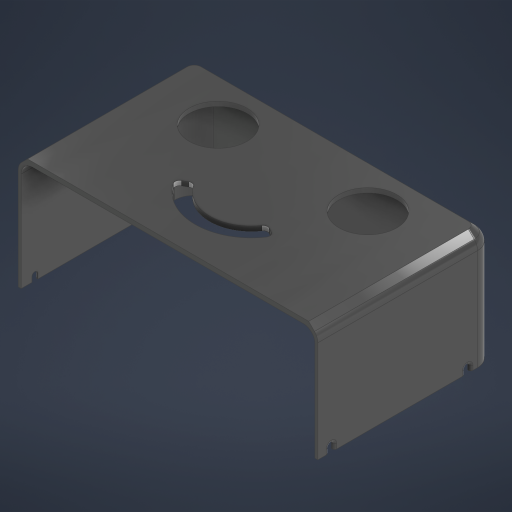
# Autodesk Inventor part: Mixer and nozzle cover
Saved by Autodesk Inventor 2024 (Build 280153000, 153)
## iProperties
Created: 2024-11-27
Part Number: Mixer and nozzle cover
Material: Generic
Document SubType Name: Modeling
Designer: Vincent Larson
Density: 1 g/cm^3
Appearance: Default
Author: Vincent Larson
## iProperties of the stored document Mixer and nozzle cover_3DPrint.ipt
Created: 2024-11-27
Part Number: Mixer and nozzle cover_3DPrint
Material: Generic
Document SubType Name: Modeling
Designer: Vincent Larson
Density: 1 g/cm^3
Appearance: Default
Author: Vincent Larson
Autodesk Inventor part; units mm, degrees
ref_plane "YZ Plane" through (0, 0, 0) normal (1, 0, 0) x (0, 1, 0)
ref_plane "XZ Plane" through (0, 0, 0) normal (0, 1, 0) x (-1, 0, 0)
ref_plane "XY Plane" through (0, 0, 0) normal (0, 0, 1) x (1, 0, 0)
sketch "Sketch1" plane through (0, 0, 0) normal (0, 1, 0) x (-1, 0, 0)
  line L0 (0, 0) -> (0, -70.91)
  line L1 (0, 0) -> (-126.245, 0)
  line L2 (-126.245, 0) -> (-126.245, -70.91)
  line L3 (-126.245, -70.91) -> (0, -70.91)
  line L4 (0, -70.91) -> (0, 0)
  line L5 (-126.245, -70.91) -> (-118.245, -70.91)
  line L6 (-118.245, -70.91) -> (-118.245, -62.91)
  circle A0 centre (-118.245, -62.91) radius 8
  line L7 (0, 0) -> (-8, 0)
  line L8 (-8, 0) -> (-8, -8)
  line L9 (-8, -8) -> (0, -8)
  line L10 (0, -8) -> (0, 0)
  circle A1 centre (-8, -62.91) radius 8
  line L11 (0.5, 0) -> (0.5, -70.91)
  circle A2 centre (-8, -62.91) radius 8.5
  line L12 (-126.245, -71.41) -> (0.5, -71.41)
  line L13 (0.5, -71.41) -> (0.5, 0)
  circle A3 centre (-118.245, -62.91) radius 8.5
  line L14 (-126.745, -70.91) -> (-126.745, 0.5)
  line L15 (-126.745, 0.5) -> (0, 0.5)
  line L16 (-8.5, 0.5) -> (0.5, 0.5)
  line L17 (0.5, 0.5) -> (0.5, -8.5)
  line L18 (0.5, -8.5) -> (-8.5, -8.5)
  line L19 (-8.5, -8.5) -> (-8.5, 0.5)
  line L20 (0.5, 0.5) -> (1.77, 0.5)
  line L21 (-126.745, -71.41) -> (-124.2953, -71.41)
  line L22 (-126.745, -69.4465) -> (-126.745, -71.41)
  circle A4 centre (-126.745, -71.41) radius 0.635
  line L23 (-127.38, -72.045) -> (1.77, -72.045)
  line L24 (1.77, -72.045) -> (1.77, 0.5)
  line L25 (1.77, 0.5) -> (-127.38, 0.5)
  line L26 (-127.38, 0.5) -> (-127.38, -72.045)
  line L27 (1.77, 0.5) -> (0.5, 0.5)
  line L28 (0.5, 0.5) -> (0.5, 3.5)
  line L29 (0.5, 3.5) -> (1.77, 3.5)
  line L30 (1.77, 3.5) -> (1.77, 0.5)
  line L31 (-126.745, 0.5) -> (-128.015, 0.5)
  line L32 (-128.015, 0.5) -> (-128.015, -72.045)
  line L33 (-128.015, -72.045) -> (-126.745, -72.045)
  line L34 (-126.745, -72.045) -> (-126.745, 0.5)
  line L35 (1.77, -71.41) -> (-128.015, -71.41)
  line L36 (-128.015, -71.41) -> (-128.015, -72.68)
  line L37 (-128.015, -72.68) -> (1.77, -72.68)
  line L38 (1.77, -72.68) -> (1.77, -71.41)
  line L39 (-126.745, 0.5) -> (-128.015, 0.5)
  line L40 (-128.015, 0.5) -> (-128.015, 3.5)
  line L41 (-128.015, 3.5) -> (-126.745, 3.5)
  line L42 (-126.745, 3.5) -> (-126.745, 0.5)
  point P0 (0.5, -62.91)
  point P1 (-8, -71.41)
  point P2 (-118.245, -71.41)
  point P3 (-126.745, -62.91)
  point P4 (-126.745, 0.5)
  point P5 (0.5, 0.5)
  point P6 (-126.745, 0.5)
  point P7 (1.77, -72.045)
  dimension "d0" = 70.91
  dimension "d1" = 126.245
  dimension "d2" = 8
  dimension "d3" = 8
  dimension "d4" = 8
  dimension "d5" = 8
  dimension "d6" = 0.5
  dimension "d7" = 0.5
  dimension "d8" = 0.5
  dimension "d9" = 0.5
  dimension "d10" = 0.5
  dimension "d11" = 0.5
  dimension "d12" = 1.27
  dimension "d13" = 1.27
  dimension "d16" = 3
  dimension "d17" = 1.27
  dimension "d18" = 1.27
  constraints: 86 end point, 18 parallel, 9 perpendicular, 8 horizontal, 8 point on line, 5 centre point, 2 coincident, 2 tangent, 1 collinear, 1 vertical, 5 other
  measures "d0" distance of L0.start L0.end
  measures "d1" distance of L3.end L2.end
  measures "d2" distance of L2.end L5.end
  measures "d3" distance of L5.end L6.end
  measures "d4" distance of L9.end L8.end
  measures "d5" distance of L8.end L7.end
  measures "d6" distance between parallel lines of L0 L11
  measures "d7" radial gap between concentric circles of A1 A2
  measures "d8" distance between parallel lines of L3 L12
  measures "d9" radial gap between concentric circles of A0 A3
  measures "d10" distance between parallel lines of L2 L14
  measures "d11" distance between parallel lines of L7 L16
  measures "d12" distance of L16.end L20.end
  measures "d13" diameter of A4
  measures "d16" distance of L27.end L28.end
  measures "d17" distance of L33.end L32.end
  measures "d18" distance of L36.end L35.end
extrude "Extrusion1" add sketch "Sketch1" along normal blind 50 contours L11 L17 L20 L24 L35 L13 | L11 L13 L12 A2 L3 L0 | L14 A4 L26 L25 | L25 L31 L40 L41 L42 | L0 L3 A2 | L12 L35 L24 L23 A4 | L28 L29 L30 L20 | A3 L2 L3 L12 A4 L14 | L26 L35 L32 L31 | A3 L3 L2 | L35 L34 A4 | A4 L23 L26 | A4 L14 L22 L35 | L26 L33 L32 L35 | A4 L12 L21 L22 L14 | L34 L21 L12 A4 | L23 L38 L37 L36 L33
sketch "Sketch2" plane through (0, 50, 0) normal (0, 1, 0) x (1, 0, 0)
  line L0 (-1.77, 72.68) -> (-1.77, -3.5) projected
  line L1 (128.015, 72.68) -> (-1.77, 72.68) projected
  line L2 (-1.77, -3.5) -> (128.015, -3.5)
  line L3 (128.015, -3.5) -> (128.015, 72.68)
  line L4 (128.015, 72.68) -> (-1.77, 72.68)
  line L5 (-1.77, 72.68) -> (-1.77, -3.5)
  point P0 (0, 0)
  constraints: 8 end point, 2 parallel, 1 horizontal, 1 perpendicular
extrude "Extrusion2" add sketch "Sketch2" against normal blind 2
fillet "Fillet1" radius 7 2 edges at (-1.77, 25, -72.68) (128.015, 25, -72.68)
sketch "Sketch3" plane through (0, 50, 0) normal (0, 1, 0) x (1, 0, 0)
  line L0 (126.745, 62.91) -> (126.745, -3.5) projected
  line L1 (126.745, 9.2311) -> (126.745, -20.0189)
  line L2 (126.745, 9.2311) -> (97.495, 9.2311)
  line L3 (128.015, -3.5) -> (128.015, 65.68) projected
  line L4 (126.745, 9.2311) -> (155.995, 9.2311) construction
  line L5 (97.495, 9.2311) -> (97.495, 85.2679)
  line L6 (121.015, 72.68) -> (5.23, 72.68) projected
  line L7 (97.495, 72.68) -> (97.495, 41.88)
  line L8 (77.495, 21.88) -> (117.495, 21.88)
  line L9 (117.495, 21.88) -> (117.495, 61.88)
  line L10 (117.495, 61.88) -> (77.495, 61.88)
  line L11 (77.495, 61.88) -> (77.495, 21.88)
  line L12 (77.495, 21.88) -> (117.495, 61.88) construction
  line L13 (117.495, 21.88) -> (77.495, 61.88) construction
  line L14 (117.495, 61.88) -> (113.495, 61.88)
  line L15 (113.495, 61.88) -> (113.495, 57.88)
  line L16 (113.495, 57.88) -> (117.495, 57.88)
  line L17 (117.495, 57.88) -> (117.495, 61.88)
  circle A0 centre (113.495, 57.88) radius 4
  circle A1 centre (113.495, 57.88) radius 1.6
  circle A2 centre (113.495, 25.88) radius 1.6
  circle A3 centre (81.495, 25.88) radius 1.6
  circle A4 centre (81.495, 57.88) radius 1.6
  circle A5 centre (97.495, 41.88) radius 19
  point P0 (0, 0)
  dimension "d22" = 29.25
  dimension "d23" = 29.25
  dimension "d24" = 180
  dimension "d25" = 30.8
  dimension "d26" = 40
  dimension "d27" = 40
  dimension "d28" = 4
  dimension "d29" = 4
  dimension "d30" = 3.2
  dimension "d31" = 3.2
  dimension "d32" = 3.2
  dimension "d33" = 3.2
  dimension "d34" = 38
  constraints: 30 end point, 7 point on line, 5 centre point, 4 parallel, 4 perpendicular, 3 coincident, 3 horizontal, 2 collinear, 2 midpoint, 1 vertical alignment, 2 other
  measures "d22" distance of L1.start L1.end
  measures "d23" distance of L1.start L2.end
  measures "d24" angle of L2 L4
  measures "d25" distance of L7.start L7.end
  measures "d26" distance of L10.end L9.end
  measures "d27" distance of L9.end L8.end
  measures "d28" distance of L16.end L15.end
  measures "d29" distance of L15.end L14.end
  measures "d30" diameter of A1
  measures "d31" diameter of A2
  measures "d32" diameter of A3
  measures "d33" diameter of A4
  measures "d34" diameter of A5
extrude "Extrusion3" cut sketch "Sketch3" against normal blind 12.2875 contours A5 L5 | L5 A5 A0 | A5 A0 | A1 L15 L16 | L16 L15 A1 | A2 | A3 | A4
fillet "Fillet3" radius 5 5 edges at (1.9896, 48, -68.9204) (-0.5, 48, 2) (124.2554, 48, -68.9204) (126.745, 48, -29.705) (63.1225, 48, -71.41)
chamfer "Chamfer1" distance 4 angle 45 5 edges at (128.015, 50, -31.09) (125.9647, 50, -70.6297) (63.1225, 50, -72.68) (0.2803, 50, -70.6297) (-1.77, 50, -31.09)
fillet "Fillet4" radius 5 5 edges at (63.1225, 46, -72.68) (0.2803, 46, -70.6297) (-1.77, 46, -31.09) (128.015, 46, -31.09) (125.9647, 46, -70.6297)
sketch "Sketch4" plane through (128.015, 0, 3.5) normal (1, 0, 0) x (0, 0, -1)
  line L0 (0, 0) -> (0, 43) projected
  line L1 (0, 0) -> (5.905, 0)
  line L2 (66.41, 0) -> (0, 0) projected
  line L3 (0, 0) -> (64.91, 0)
  line L4 (0, 0) -> (64.91, 0) construction
  line L5 (64.91, 0) -> (64.91, 1.65)
  line L6 (64.91, 0) -> (66.56, 0) construction
  line L7 (5.905, 0) -> (5.905, 1.853)
  circle A0 centre (5.905, 1.853) radius 1.27
  circle A1 centre (64.91, 1.65) radius 1.27
  line L8 (64.91, 0.38) -> (64.91, 0)
  line L9 (64.91, 1.65) -> (64.91, 1.95)
  line L10 (5.905, 1.853) -> (5.905, 2.153)
  line L11 (5.905, 2.153) -> (5.905, -2.5313) construction
  line L12 (4.635, 2.153) -> (4.635, -2.5313)
  line L13 (7.175, -2.5313) -> (7.175, 2.153)
  arc A2 (7.175, 2.153) -> (4.635, 2.153) centre (5.905, 2.153) ccw
  arc A3 (4.635, -2.5313) -> (7.175, -2.5313) centre (5.905, -2.5313) ccw
  line L14 (64.91, 1.95) -> (64.91, -2.4175) construction
  line L15 (63.6436, 1.95) -> (63.6436, -2.4175)
  line L16 (66.1764, -2.4175) -> (66.1764, 1.95)
  arc A4 (66.1764, 1.95) -> (63.6436, 1.95) centre (64.91, 1.95) ccw
  arc A5 (63.6436, -2.4175) -> (66.1764, -2.4175) centre (64.91, -2.4175) ccw
  point P0 (3.5, 0)
  point P1 (5.905, -0.1892)
  point P2 (64.91, -0.2337)
  dimension "d50" = 2.54
  dimension "d43" = 5.905
  dimension "d44" = 64.91
  dimension "d45" = 0
  dimension "d46" = 1.65
  dimension "d47" = 90
  dimension "d48" = 1.853
  dimension "d49" = 2.54
  dimension "d51" = 0.3
  dimension "d52" = 0.3
  constraints: 34 end point, 8 point on circle, 8 tangent, 5 centre point, 4 point on line, 4 vertical, 2 coincident, 2 collinear, 2 equal length, 2 horizontal, 2 midpoint, 2 parallel, 1 vertical alignment, 2 other
  measures "d43" distance of L0.start L1.end
  measures "d44" distance of L0.start L3.end
  measures "d45" distance between parallel lines of L3 L4
  measures "d46" distance of L4.end L5.end
  measures "d47" angle of L6 L5
  measures "d48" distance of L1.end L7.end
  measures "d49" diameter of A0
  measures "d51" distance of L9.start L9.end
  measures "d52" distance of L10.start L10.end
extrude "Extrusion4" cut sketch "Sketch4" against normal blind 143.2875 contours L12 A0 L7 L1 | L1 L2 L13 A3 L12 | L7 A0 L13 L2 | L12 A2 L13 A0 | A0 | L16 A5 L15 L2 | L2 L5 A1 L16 | L2 L15 A1 L5 | A1 L15 L16 | A1 L15 A4 L16
fillet "Fillet5" radius 1 12 edges at (128.015, 0.975, -62.6764) (128.015, 0.975, -60.1436) (128.015, 3.2164, -61.41) (128.015, 1.0765, -3.675) (128.015, 1.0765, -1.135) (128.015, 3.423, -2.405) (-1.77, 1.0765, -1.135) (-1.77, 1.0765, -3.675) (-1.77, 3.423, -2.405) (-1.77, 0.975, -60.1436) (-1.77, 0.975, -62.6764) (-1.77, 3.2164, -61.41)
sketch "Sketch5" plane through (121.015, 0, -72.68) normal (0, 0, -1) x (-1, 0, 0)
  line L0 (0, 0) -> (115.785, 0) projected
  line L1 (57.8925, 0) -> (57.8925, 61.1209)
  line L2 (57.8925, 0) -> (57.8925, 8)
  line L3 (57.8925, 4) -> (72.8925, 4)
  line L4 (72.8925, 4) -> (42.8925, 4)
  circle A0 centre (72.8925, 4) radius 4
  circle A1 centre (57.8925, 4) radius 4
  circle A2 centre (42.8925, 4) radius 4
  line L5 (72.8925, 4) -> (42.8925, 4) construction
  line L6 (72.8925, 8.5763) -> (42.8925, 8.5763)
  line L7 (42.8925, -0.5763) -> (72.8925, -0.5763)
  arc A3 (72.8925, -0.5763) -> (72.8925, 8.5763) centre (72.8925, 4) ccw
  arc A4 (42.8925, 8.5763) -> (42.8925, -0.5763) centre (42.8925, 4) ccw
  line L8 (38.3162, 4) -> (77.4688, 4)
  line L9 (77.4688, 4) -> (77.4688, -4.4635)
  line L10 (77.4688, -4.4635) -> (38.3162, -4.4635)
  line L11 (38.3162, -4.4635) -> (38.3162, 4)
  circle A5 centre (57.8925, 4) radius 7
  circle A6 centre (72.8925, 4) radius 7
  circle A7 centre (42.8925, 4) radius 7
  line L12 (72.8925, 4) -> (42.8925, 4) construction
  line L13 (72.8925, 11) -> (42.8925, 11)
  line L14 (42.8925, -3) -> (72.8925, -3)
  arc A8 (72.8925, -3) -> (72.8925, 11) centre (72.8925, 4) ccw
  arc A9 (42.8925, 11) -> (42.8925, -3) centre (42.8925, 4) ccw
  line L15 (79.8925, 4) -> (35.8925, 4)
  line L16 (35.8925, 4) -> (35.8925, -6.7198)
  line L17 (35.8925, -6.7198) -> (79.8925, -6.7198)
  line L18 (79.8925, -6.7198) -> (79.8925, 4)
  point P0 (121.015, 0)
  dimension "d56" = 8
  dimension "d57" = 15
  dimension "d58" = 30
  dimension "d64" = 14
  constraints: 40 end point, 10 point on circle, 10 tangent, 9 centre point, 6 coincident, 6 parallel, 4 midpoint, 3 horizontal, 2 collinear, 2 perpendicular, 2 point on line, 1 vertical, 1 vertical alignment, 2 other
  measures "d56" distance of L1.start L2.end
  measures "d57" distance of L3.start L3.end
  measures "d58" distance of L3.end L4.end
  measures "d64" diameter of A5
extrude "Extrusion5" cut sketch "Sketch5" against normal blind 143.2875
sketch "Sketch6" plane through (121.015, 43.9289, -72.68) normal (0, 0, -1) x (-1, 0, 0)
  line L0 (107.9273, -39.9289) -> (92.2741, -39.9289) construction
  line L1 (107.9273, -44.5052) -> (92.2741, -44.5052)
  line L2 (92.2741, -35.3527) -> (107.9273, -35.3527)
  arc A0 (107.9273, -44.5052) -> (107.9273, -35.3527) centre (107.9273, -39.9289) ccw
  arc A1 (92.2741, -35.3527) -> (92.2741, -44.5052) centre (92.2741, -39.9289) ccw
  line L3 (87.6978, -39.9289) -> (112.5036, -39.9289)
  line L4 (112.5036, -39.9289) -> (112.5036, -53.2289)
  line L5 (112.5036, -53.2289) -> (87.6978, -53.2289)
  line L6 (87.6978, -53.2289) -> (87.6978, -39.9289)
  point P0 (121.015, -43.9289)
  point P1 (100.1007, -39.9289)
  constraints: 16 end point, 5 point on circle, 4 tangent, 3 parallel, 2 centre point, 2 horizontal, 1 midpoint, 1 perpendicular
extrude "Extrusion6" cut sketch "Sketch6" against normal blind 143.2875
fillet "Fillet7" radius 1 10 edges at (20.9143, 8.5763, -72.68) (9.8518, 7.2359, -72.68) (8.5114, 2, -72.68) (33.3172, 2, -72.68) (31.9768, 7.2359, -72.68) (43.1728, 8.9497, -72.68) (41.1225, 2, -72.68) (83.0722, 8.9497, -72.68) (85.1225, 2, -72.68) (63.1225, 11, -72.68)
fillet "Fillet8" radius 1 10 edges at (33.3172, 2, -71.41) (20.9143, 8.5763, -71.41) (9.8518, 7.2359, -71.41) (8.5114, 2, -71.41) (31.9768, 7.2359, -71.41) (83.0722, 8.9497, -71.41) (85.1225, 2, -71.41) (43.1728, 8.9497, -71.41) (41.1225, 2, -71.41) (63.1225, 11, -71.41)
sketch "Sketch7" plane through (0, 50, 0) normal (0, 1, 0) x (1, 0, 0)
  line L0 (124.015, -3.5) -> (126.5505, -3.5) projected
  line L1 (2.23, 68.68) -> (124.015, 68.68)
  line L2 (124.015, 68.68) -> (124.015, -3.5)
  line L3 (124.015, -3.5) -> (2.23, -3.5)
  line L4 (2.23, -3.5) -> (2.23, 68.68)
  line L5 (124.015, -3.5) -> (63.1225, -3.5)
  line L6 (121.745, -3.5) -> (4.5, -3.5) projected
  line L7 (63.1225, -3.5) -> (2.23, -3.5)
  line L8 (32.6762, -3.5) -> (32.6762, 68.68)
  circle A0 centre (97.495, 41.88) radius 19 projected
  line L9 (97.495, 41.88) -> (32.6762, 41.88)
  circle A1 centre (32.6762, 41.88) radius 20.25
  point P0 (0, 0)
  dimension "d67" = 40.5
  constraints: 16 end point, 3 perpendicular, 2 midpoint, 2 parallel, 2 point on line, 1 centre point, 1 coincident, 1 collinear, 1 horizontal
  measures "d67" diameter of A1
extrude "Extrusion7" cut sketch "Sketch7" against normal blind 12.2875 contours A1 L9 L8 | L8 A1 | L9 A1 L8
sketch "Sketch8" plane through (0, 50, 0) normal (0, 1, 0) x (1, 0, 0)
  arc A0 (32.6762, 11.2053) -> (97.495, 11.2053) centre (65.0856, 68.6468) ccw
  line L0 (32.6762, 11.2053) -> (97.495, 11.2053) construction
  line L1 (32.6762, 11.2053) -> (97.495, 11.2053) construction
  arc A1 (32.6762, 11.2053) -> (97.495, 11.2053) centre (65.0856, 103.0763) ccw
  arc A2 (32.6762, 11.2053) -> (97.495, 11.2053) centre (65.0856, 52.4718) ccw
  point P0 (0, 0)
  dimension "d70" = 0
  constraints: 6 point on circle, 4 end point, 3 centre point, 1 collinear, 1 horizontal
  measures "d70" distance between parallel lines of L0 L1
extrude "Extrusion8" cut sketch "Sketch8" against normal blind 9.1125
fillet "Fillet9" radius 0.5 2 edges at (32.6762, 49, -11.2053) (97.495, 49, -11.2053)
sketch "Sketch10" plane through (0, 50, 0) normal (0, 1, 0) x (1, 0, 0)
  circle A0 centre (81.495, 25.88) radius 1.6 projected
  circle A1 centre (81.495, 25.88) radius 2.7243
  circle A2 centre (113.495, 57.88) radius 1.6 projected
  circle A3 centre (113.495, 57.88) radius 2.7174
  circle A4 centre (81.495, 57.88) radius 1.6 projected
  circle A5 centre (81.495, 57.88) radius 2.7174
  circle A6 centre (113.495, 25.88) radius 1.6 projected
  circle A7 centre (113.495, 25.88) radius 3.1594
  point P0 (0, 0)
  constraints: 4 centre point, 4 coincident
extrude "Extrusion9" add sketch "Sketch10" against normal up to surface (2 mm away) contours A0 | A1 | A2 | A3 | A4 | A5 | A6 | A7
sketch "Sketch14" plane through (-1.77, 0, 3.5) normal (-1, 0, 0) x (0, 0, 1)
  line L0 (-74.7155, 47.4645) -> (-72.18, 50) projected
  line L1 (-72.18, 50) -> (-77.4448, 44.7352)
  arc A0 (-74.7155, 47.4645) -> (-76.18, 43.9289) centre (-71.18, 43.9289) ccw projected
  circle A1 centre (-71.18, 43.9289) radius 5
  line L2 (-72.18, 45.5127) -> (-80.544, 45.5127)
  line L3 (-80.544, 45.5127) -> (-80.544, 49.5156)
  line L4 (-80.544, 49.5156) -> (-72.18, 49.5156)
  line L5 (-72.18, 49.5156) -> (-72.18, 45.5127)
  point P0 (-3.5, 0)
  point P1 (-75.9225, 45.5127)
  point P2 (-72.6644, 49.5156)
  constraints: 10 end point, 2 parallel, 1 centre point, 1 coincident, 1 collinear, 1 horizontal, 1 perpendicular
extrude "Extrusion13" cut sketch "Sketch14" against normal blind 140.2875 contours L1 L2 L3 L4 L0 | A0 L2 L1
sketch "Sketch15" plane through (0, 50, 0) normal (0, 1, 0) x (1, 0, 0)
  circle A0 centre (97.495, 41.88) radius 19 projected
  circle A1 centre (97.495, 41.88) radius 19
  line L0 (97.495, 41.88) -> (54.4425, 79.3182)
  line L1 (97.495, 41.88) -> (154.5488, 41.88) construction
  line L2 (97.495, 41.88) -> (140.044, 3.5822)
  line L3 (97.495, 41.88) -> (154.7413, 41.88) construction
  line L4 (97.495, 41.88) -> (117.4939, 23.8792)
  line L5 (97.495, 41.88) -> (74.4949, 61.8807)
  circle A2 centre (74.4949, 61.8807) radius 2.25
  circle A3 centre (117.4939, 23.8792) radius 2.25
  point P0 (0, 0)
  dimension "d105" = 138.99
  dimension "d106" = 41.99
  dimension "d107" = 26.907
  dimension "d108" = 30.48
  dimension "d109" = 4.5
  dimension "d110" = 4.5
  constraints: 12 end point, 3 centre point, 3 coincident, 2 equal length, 2 horizontal, 2 point on line
  measures "d105" angle of L1 L0
  measures "d106" angle of L2 L3
  measures "d107" distance of L0.start L4.end
  measures "d108" distance of L0.start L5.end
  measures "d109" diameter of A2
  measures "d110" diameter of A3
extrude "Extrusion14" cut sketch "Sketch15" against normal blind 10.525 contours A2 L0 | L0 A2 | A3 L2 | L2 A3
sketch "Sketch17" plane through (0, 50, 0) normal (0, 1, 0) x (1, 0, 0)
  circle A0 centre (97.495, 41.88) radius 19 projected
  circle A1 centre (97.495, 41.88) radius 19
  circle A2 centre (97.495, 41.88) radius 17.5
  circle A3 centre (74.3414, 60.6185) radius 5.462
  circle A4 centre (78.495, 60.6185) radius 7.5644
  circle A5 centre (115.7578, 21.8617) radius 6.4868
  point P0 (0, 0)
  dimension "d118" = 35
  constraints: 5 centre point, 2 coincident
  measures "d118" diameter of A2
extrude "Extrusion16" add sketch "Sketch17" against normal up to surface (2 mm away) contours A0 | A3 A4 | A3 A4 | A5 picked at (73.9195, 60.6185) picked at (83.9041, 61.2083)
sketch "Sketch18" plane through (0, 50, 0) normal (0, 1, 0) x (1, 0, 0)
  circle A0 centre (97.495, 41.88) radius 17.5 projected
  circle A1 centre (97.495, 41.88) radius 17.5
  circle A2 centre (32.6762, 41.88) radius 20.25 projected
  circle A3 centre (32.6762, 41.88) radius 20.25
  circle A4 centre (32.6762, 41.88) radius 17.5
  point P0 (0, 0)
  constraints: 3 centre point, 3 coincident
extrude "Extrusion17" add sketch "Sketch18" against normal up to surface (2 mm away) contours A2
sketch "Sketch19" plane through (0, 50, 0) normal (0, 1, 0) x (1, 0, 0)
  line L0 (8.9671, 64.4302) -> (117.1286, 64.4302)
  line L1 (117.1286, 64.4302) -> (117.1286, 14.3842)
  line L2 (117.1286, 14.3842) -> (8.9671, 14.3842)
  line L3 (8.9671, 14.3842) -> (8.9671, 64.4302)
  point P0 (0, 0)
  constraints: 8 end point, 2 parallel, 1 horizontal, 1 perpendicular
extrude "Extrusion18" add sketch "Sketch19" against normal up to surface (2 mm away)
sketch "Sketch20" plane through (0, 50, 0) normal (0, 1, 0) x (1, 0, 0)
  line L0 (2.23, -3.5) -> (2.23, 65.68) projected
  line L1 (2.23, 38.2427) -> (124.015, 38.2427)
  line L2 (124.015, 65.68) -> (124.015, -3.5) projected
  line L3 (63.1225, 38.2427) -> (63.1225, 5.6761)
  arc A0 (35.6778, 10.201) -> (94.4934, 10.201) centre (65.0856, 103.0763) ccw projected
  line L4 (23.291, 16.9801) -> (104.6193, 16.9801)
  line L5 (104.6193, 16.9801) -> (104.6193, -1.8069)
  line L6 (104.6193, -1.8069) -> (23.291, -1.8069)
  line L7 (23.291, -1.8069) -> (23.291, 16.9801)
  point P0 (0, 0)
  constraints: 12 end point, 2 horizontal, 2 parallel, 2 perpendicular, 2 point on line, 1 midpoint, 1 point on circle
extrude "Extrusion19" add sketch "Sketch20" against normal up to surface (2 mm away)
sketch "Sketch21" plane through (0, 50, 0) normal (0, 1, 0) x (1, 0, 0)
  line L0 (121.745, -3.5) -> (4.5, -3.5) projected
  line L1 (63.1225, -3.5) -> (63.1225, 68.68)
  line L2 (5.23, 68.68) -> (121.015, 68.68) projected
  line L3 (63.1225, 32.59) -> (-1.77, 32.59)
  line L4 (-1.77, 65.68) -> (-1.77, -3.5) projected
  line L5 (-1.77, 32.59) -> (128.015, 32.59)
  line L6 (128.015, 4.675) -> (128.015, 59.1436) projected
  line L7 (63.1225, 32.59) -> (63.1225, -3.5)
  line L8 (63.1225, 32.59) -> (63.1225, 68.68)
  line L9 (63.1225, 32.59) -> (-1.77, 32.59)
  line L10 (63.1225, 32.59) -> (128.015, 32.59)
  line L11 (95.5687, 32.59) -> (63.1225, 50.635)
  line L12 (63.1225, 50.635) -> (30.6762, 32.59)
  line L13 (63.1225, 32.59) -> (46.8994, 41.6125)
  line L14 (63.1225, 32.59) -> (79.3456, 41.6125)
  line L15 (63.1225, 32.59) -> (95.5687, 50.635)
  line L16 (95.5687, 50.635) -> (63.1225, 32.59)
  line L17 (63.1225, 32.59) -> (30.6762, 50.635)
  circle A0 centre (30.6762, 50.635) radius 12.5
  circle A1 centre (95.5687, 50.635) radius 12.5
  circle A2 centre (63.1225, 32.59) radius 18.045
  line L18 (63.1225, 32.59) -> (30.6762, 32.59)
  line L19 (46.8994, 32.59) -> (30.6762, 32.59)
  line L20 (38.7878, 32.59) -> (38.7878, 46.1237)
  circle A3 centre (63.1225, 32.59) radius 24.3347
  line L21 (90.7677, 47.9649) -> (21.7602, 9.5863)
  line L22 (30.6762, 50.635) -> (102.9145, 10.4596)
  point P0 (0, 0)
  point P1 (47.3523, 23.8194)
  point P2 (41.8555, 20.7624)
  point P3 (84.3895, 20.7624)
  point P4 (78.8927, 23.8194)
  dimension "d127" = 25
  dimension "d128" = 25
  constraints: 38 end point, 10 midpoint, 9 point on line, 5 collinear, 4 coincident, 3 centre point, 3 perpendicular, 3 other
  measures "d127" diameter of A0
  measures "d128" diameter of A1
extrude "Extrusion20" cut sketch "Sketch21" against normal blind 15.4 contours A2 L22 A3 L1 | L1 A3 L21 A2 | A0 L20 L17 | L17 L20 A0 | A1
fillet "Fillet15" radius 2 4 edges at (47.3523, 49, -23.8194) (78.8927, 49, -23.8194) (84.3895, 49, -20.7624) (41.8555, 49, -20.7624)
body "Solid1"
